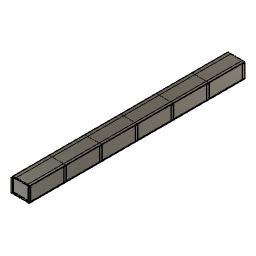
Model v3 (Autodesk Fusion 360 design; units mm, degrees)
Autodesk Fusion 360 part; units mm, degrees
sketch "Sketch1" plane through (0, 0, 0) normal (0, 1, 0) x (1, 0, 0)
  line L0 (-10, -88.81) -> (90, -88.81)
  line L1 (90, -88.81) -> (90, -87.54)
  line L2 (90, -87.54) -> (-10, -87.54)
  line L3 (-10, -87.54) -> (-10, -88.81)
  line L4 (6.26, -87.54) -> (-10, -87.54)
  line L5 (-10, -87.54) -> (-10, -5)
  line L6 (-10, -5) -> (6.26, -5)
  line L7 (6.26, -5) -> (6.26, -6.27)
  line L8 (6.26, -6.27) -> (-8.74, -6.27)
  line L9 (-8.74, -6.27) -> (-8.74, -86.27)
  line L10 (-8.74, -86.27) -> (6.26, -86.27)
  line L11 (6.26, -86.27) -> (6.26, -87.54)
  line L12 (40, -88.81) -> (40, -87.54) construction
  line L13 (73.74, -87.54) -> (90, -87.54)
  line L14 (73.74, -86.27) -> (73.74, -87.54)
  line L15 (88.74, -86.27) -> (73.74, -86.27)
  line L16 (90, -87.54) -> (90, -5)
  line L17 (88.74, -6.27) -> (88.74, -86.27)
  line L18 (73.74, -5) -> (73.74, -6.27)
  line L19 (73.74, -6.27) -> (88.74, -6.27)
  line L20 (90, -5) -> (73.74, -5)
  line L21 (-15.1597, -88.81) -> (104, -88.81) construction
  line L22 (90, -88.81) -> (90, -90.08)
  line L23 (73.74, -90.08) -> (90, -90.08)
  line L24 (-10, -88.81) -> (90, -88.81)
  line L25 (90, -90.08) -> (-10, -90.08)
  line L26 (-10, -90.08) -> (-10, -88.81)
  line L27 (-10, -5) -> (90, -5)
  line L28 (90, -5) -> (90, -3.73)
  line L29 (90, -3.73) -> (-10, -3.73)
  line L30 (-10, -3.73) -> (-10, -5)
  line L31 (-14.7091, -3.73) -> (97, -3.73) construction
  line L32 (-10, -2.46) -> (90, -2.46)
  line L33 (-10, -3.73) -> (-10, -2.46)
  line L34 (90, -2.46) -> (90, -3.73)
  dimension "d1" = 1.27
  dimension "d2" = 100
  dimension "d3" = 1.27
  dimension "d4" = 1.27
  dimension "d5" = 1.26
  dimension "d6" = 80
  dimension "d7" = 15
  dimension "d8" = 100
  dimension "d9" = 1.27
  dimension "d12" = 15
  dimension "d13" = 15
  constraint horizontal L0
  constraint vertical L1
  constraint horizontal L2
  constraint vertical L3
  constraint horizontal L4
  constraint perpendicular L4 L5
  constraint perpendicular L5 L6
  constraint perpendicular L6 L7
  constraint perpendicular L7 L8
  constraint perpendicular L8 L9
  constraint perpendicular L7 L10
  constraint parallel L5 L11
  constraint collinear L2 L4
  constraint collinear L3 L5
  constraint midpoint L0 L12.start
  constraint midpoint L2 L12.end
  constraint symmetric L4.start L12 L13.start
  constraint symmetric L2.end L12 L1.end
  constraint symmetric L5.end L12 L16.end
  constraint symmetric L6.end L12 L18.start
  constraint symmetric L7.end L12 L18.end
  constraint symmetric L8.end L12 L17.start
  constraint symmetric L9.end L12 L15.start
  constraint symmetric L10.end L12 L14.start
  constraint perpendicular L3 L21
  constraint symmetric L0.start L21 L3.end
  constraint symmetric L0.end L21 L1.start
  constraint symmetric L1.end L21 L22.end
  constraint symmetric L2.end L21 L25.end
  constraint symmetric L13.start L21 L23.start
  constraint horizontal L27
  constraint vertical L28
  constraint horizontal L29
  constraint vertical L30
  constraint collinear L6 L27
  constraint collinear L5 L30
  constraint parallel L27 L31
  constraint symmetric L5.end L31 L32.start
  constraint symmetric L16.end L31 L32.end
  constraint symmetric L28.end L31 L29.start
  constraint symmetric L29.end L31 L30.start
  measures "d1" distance of L0 L2
  measures "d2" distance of L1 L3
  measures "d3" distance of L4 L10
  measures "d4" distance of L6 L8
  measures "d5" distance of L5 L9
  measures "d6" distance of L8 L10
  measures "d7" distance of L9 L11
  measures "d8" distance of L28 L30
  measures "d9" distance of L27 L29
  measures "d12" distance of L7 L9
  measures "d13" distance of L17 L18
extrude "Extrude1" add sketch "Sketch1" along normal blind 1270 contours L0 L1 L2 L3 L4 L13 L24 | L0 L22 L23 L24 L25 L26 | L2 L4 L5 L6 L7 L8 L9 L10 L11 L27 | L2 L13 L14 L15 L16 L17 L18 L19 L20 L27 | L6 L20 L27 L28 L29 L30 | L29 L32 L33 L34 makes body 1
sketch "Sketch1 (2)" plane through (0, 0, 0) normal (0, 0, 1) x (1, 0, 0) in component "Middle Plate"
  line L0 (-41.54, 20) -> (61, 20)
  line L1 (61, 20) -> (61, 5)
  line L2 (61, 5) -> (59.73, 5)
  line L3 (59.73, 5) -> (59.73, 18.73)
  line L4 (59.73, 18.73) -> (-40.27, 18.73)
  line L5 (-40.27, 18.73) -> (-40.27, 5)
  line L6 (-40.27, 5) -> (-41.54, 5)
  line L7 (-41.54, 5) -> (-41.54, 20)
  dimension "d14" = 1.27
  dimension "d15" = 1.27
  dimension "d16" = 1.27
  dimension "d17" = 15
  dimension "d18" = 15
  dimension "d19" = 100
  constraint horizontal L0
  constraint perpendicular L0 L1
  constraint perpendicular L1 L2
  constraint perpendicular L2 L3
  constraint perpendicular L1 L4
  constraint perpendicular L4 L5
  constraint perpendicular L1 L6
  constraint perpendicular L0 L7
  measures "d14" distance of L5 L7
  measures "d15" distance of L1 L3
  measures "d16" distance of L0 L4
  measures "d17" distance of L0 L6
  measures "d18" distance of L0 L2
  measures "d19" distance of L3 L5
extrude "Extrude1'" add sketch "Sketch1 (2)" along normal blind 80 separate body makes body 2 in component "Middle Plate"
copy_body "Body->Comp1" bodies 1 removing the originals makes body 3 in component "Bridge"
component_pattern "component pattern"
component "Middle Plate" placed x (1, 0, 0) y (0, 1, 0) z (0, 0, 1) at (57.4871, -36.7472, -2.605)
component "Bridge" placed x (1, 0, 0) y (0, -1, 0) z (0, 0, -1) at (27.2171, -17.0172, 83.665)
component "Middle Plate" placed x (1, 0, 0) y (0, 1, 0) z (0, 0, 1) at (57.4871, -247.2088, -2.605)
component "Middle Plate" placed x (1, 0, 0) y (0, 1, 0) z (0, 0, 1) at (57.4871, -457.6705, -2.605)
component "Middle Plate" placed x (1, 0, 0) y (0, 1, 0) z (0, 0, 1) at (57.4871, -668.1322, -2.605)
component "Middle Plate" placed x (1, 0, 0) y (0, 1, 0) z (0, 0, 1) at (57.4871, -878.5938, -2.605)
component "Middle Plate" placed x (1, 0, 0) y (0, 1, 0) z (0, 0, 1) at (57.4871, -1089.0555, -2.605)
component "Middle Plate" placed x (1, 0, 0) y (0, 1, 0) z (0, 0, 1) at (57.4871, -1299.5172, -2.605)
